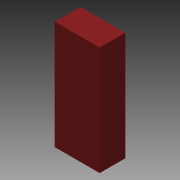
# Autodesk Inventor part: OKY2-T/10-D12
Saved by Autodesk Inventor 2015 SP1 (Build 190203100, 203)
## iProperties
Created: 2015-06-25
Part Number: OKY2-T/10-D12
Material: Generic
Document SubType Name: Modeling
Designer: Patrick
Density: 1 g/cm^3
Appearance: OKY2T10, OKY2-T_10-D12
Author: Patrick
Autodesk Inventor part; units mm, degrees
ref_plane "YZ Plane" through (0, 0, 0) normal (1, 0, 0) x (0, 1, 0)
ref_plane "XZ Plane" through (0, 0, 0) normal (0, 1, 0) x (-1, 0, 0)
ref_plane "XY Plane" through (0, 0, 0) normal (0, 0, 1) x (1, 0, 0)
sketch "OKY2T10, OKY2-T_10-D12_120" plane through (0, 0, 0) normal (0, 0, 1) x (1, 0, 0)
  line L0 (-6.85, -16.6) -> (-6.85, 16.6)
  line L1 (-6.85, 16.6) -> (6.85, 16.6)
  line L2 (6.85, 16.6) -> (6.85, -16.6)
  line L3 (6.85, -16.6) -> (-6.85, -16.6)
  constraints: 8 end point
extrude "Extrusion1" add sketch "OKY2T10, OKY2-T_10-D12_120" along normal blind 7.8
body "Solid1"
